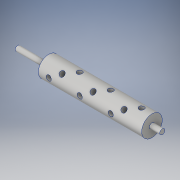
# Autodesk Inventor part: Part4
Saved by Autodesk Inventor 2019 (Build 230136000, 136)
## iProperties
Created: 2018-09-17
Part Number: Part4
Material: Aluminum 6061
Document SubType Name: Modeling
Designer: drawing
Density: 2.7 g/cm^3
Appearance: Aluminum - Flat
Mass: 160.854 g
Surface Area: 165.775 cm^2
Volume: 59.5756 cm^3
Author: drawing
Autodesk Inventor part; units mm, degrees
sketch "Sketch1" plane through (0, 0, 0) normal (0, 0, 1) x (1, 0, 0)
  line L0 (-101.6, 0) -> (-101.6, 3.175)
  line L1 (-101.6, 3.175) -> (-63.5, 3.175)
  line L2 (-63.5, 3.175) -> (-63.5, 12.7)
  line L3 (-63.5, 12.7) -> (63.5, 12.7)
  line L4 (63.5, 12.7) -> (63.5, 3.175)
  line L5 (63.5, 3.175) -> (101.6, 3.175)
  line L6 (101.6, 3.175) -> (101.6, 0)
  line L7 (101.6, 0) -> (-101.6, 0)
  point P0 (0, 0)
  point P1 (0, 0)
  dimension "d0" = 6.35
  dimension "d1" = 25.4
  dimension "d2" = 38.1
  dimension "d3" = 38.1
  dimension "d4" = 127
  constraints: 16 end point, 6 perpendicular, 2 point on line, 1 coincident, 1 midpoint, 1 vertical
  measures "d0" diameter of L5 L7
  measures "d1" diameter of L3 L7
  measures "d2" distance of L4.end L5.end
  measures "d3" distance of L0.end L1.end
  measures "d4" distance of L2.end L3.end
revolve "Revolution1" add sketch "Sketch1" angle 360 about axis through (101.6, 0, 0) along (-1, 0, 0)
ref_plane "Work Plane1" through (0, 0, 12.7) normal (0, 0, 1) x (1, 0, 0)
sketch "Sketch2" plane through (0, 0, 12.7) normal (0, 0, 1) x (1, 0, 0)
  line L0 (-63.5, -12.7) -> (-63.5, 12.7) projected
  point P0 (0, 0)
  point P1 (-50.8, 0)
  point P2 (-63.5, 0)
  dimension "d6" = 12.7
  constraints: 1 horizontal alignment, 1 midpoint
  measures "d6" distance from line of L0 point (-50.8, 0)
hole "Hole1" at (-50.8, 0, 12.7) direction (0, 0, -1) diameter 6.35 end through all
ref_plane "Work Plane3" through (0, 8.9803, 8.9803) normal (0, 0.7071, 0.7071) x (-1, 0, 0)
ref_plane "Work Plane2" through (0, 0, 0) normal (0, 0.7071, 0.7071) x (1, 0, 0)
sketch "Sketch3" plane through (0, 8.9803, 8.9803) normal (0, 0.7071, 0.7071) x (-1, 0, 0)
  line L0 (63.5, 12.7) -> (63.5, -12.7) projected
  point P0 (0, 0)
  point P1 (38.1, 0)
  point P2 (63.5, 0)
  dimension "d15" = 25.4
  constraints: 1 horizontal alignment, 1 midpoint
  measures "d15" distance from line of L0 point (38.1, 0)
hole "Hole2" at (-38.1, 8.9803, 8.9803) direction (0, -0.7071, -0.7071) diameter 6.35 end through all
ref_plane "Work Plane4" through (0, 12.7, 0) normal (0, 1, 0) x (-1, 0, 0)
sketch "Sketch4" plane through (0, 12.7, 0) normal (0, 1, 0) x (-1, 0, 0)
  line L0 (63.5, 12.7) -> (63.5, -12.7) projected
  point P0 (0, 0)
  point P1 (25.4, 0)
  point P2 (63.5, 0)
  dimension "d23" = 38.1
  constraints: 1 horizontal alignment, 1 midpoint
  measures "d23" distance from line of L0 point (25.4, 0)
hole "Hole3" at (-25.4, 12.7, 0) direction (0, -1, 0) diameter 6.35 end through all
pattern_linear "Rectangular Pattern1" count 3 spacing 38.1 along (1, 0, 0) of "Hole1", "Hole2", "Hole3"
sketch "Sketch5" plane through (101.6, 0, 0) normal (1, 0, 0) x (0, 0, -1)
  circle A0 centre (0, 0) radius 3.175 projected
  point P0 (0, 0)
extrude "Extrusion1" cut sketch "Sketch5" against normal blind 25.4
equation "\"d2\" = d3"
equation "\"d15\" = 2 * d6"
equation "\"d23\" = 3 * d6"
body "Solid1"
